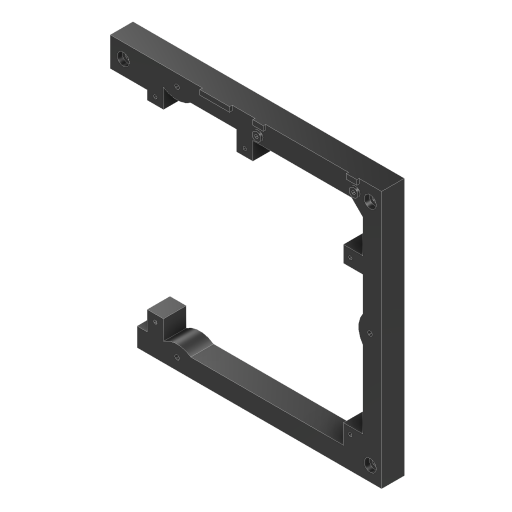
# Autodesk Inventor part: display_cover_part1
Saved by Autodesk Inventor 2023 (Build 270158000, 158)
## iProperties
Created: 2024-12-04
Part Number: display_cover_part1
Material: Polyacetátová pryskyřice, černá
Document SubType Name: Modeling
Designer: Marek
Density: 1.425 g/cm^3
Appearance: Lesklá – černá
Author: Marek
## iProperties of the stored document display_cover_part1_3D tisk.ipt
Created: 2024-12-18
Part Number: display_cover_part1_3D tisk
Material: Všeobecné
Document SubType Name: Modeling
Designer: Marek
Density: 1 g/cm^3
Appearance: Výchozí
Author: Marek
Autodesk Inventor part; units mm, degrees
ref_plane "YZ Plane" through (0, 0, 0) normal (1, 0, 0) x (0, 1, 0)
ref_plane "XZ Plane" through (0, 0, 0) normal (0, 1, 0) x (-1, 0, 0)
ref_plane "XY Plane" through (0, 0, 0) normal (0, 0, 1) x (1, 0, 0)
sketch "Náčrt1" plane through (0, 0, 0) normal (0, 0, 1) x (1, 0, 0)
  line L0 (0, 110.95) -> (0, -110.95) projected
  line L1 (-116.9, 0) -> (116.9, 0) projected
  line L2 (-83.5, 79.25) -> (83.5, 79.25)
  line L3 (83.5, -79.25) -> (-67, -79.25)
  line L4 (-83.5, 61.25) -> (-83.5, 79.25)
  line L5 (-65.5, 67.75) -> (4.25, 67.75)
  line L6 (72, 67.75) -> (72, 66.75) construction
  line L7 (-65.5, 67.75) -> (-65.5, 61.25)
  line L8 (-65.5, 61.25) -> (-83.5, 61.25)
  line L9 (-67, -67.75) -> (-67, -79.25)
  line L10 (-60.75, 65) -> (69.25, 65) construction
  line L11 (69.25, 65) -> (69.25, -65) construction
  line L12 (69.25, -65) -> (-60.75, -65) construction
  line L13 (-60.75, -65) -> (-60.75, 65) construction
  line L14 (-65.5, 61.25) -> (-60.75, 61.25)
  line L15 (-60.75, 61.25) -> (-60.75, 55.75)
  line L16 (-60.75, 55.75) -> (-50.75, 55.75)
  line L17 (-50.75, 55.75) -> (-50.75, 67.75)
  line L18 (4.25, 65) -> (4.25, 39.25) construction
  line L19 (4.25, 39.25) -> (69.25, 39.25) construction
  line L20 (4.25, 67.75) -> (4.25, 55.75)
  line L21 (4.25, 55.75) -> (-5.75, 55.75)
  line L22 (-5.75, 55.75) -> (-5.75, 67.75)
  line L23 (-67, -67.75) -> (72, -67.75)
  line L24 (83.5, 79.25) -> (83.5, -79.25)
  line L25 (-60.75, -67.75) -> (-60.75, -55.75)
  line L26 (-60.75, -55.75) -> (-50.75, -55.75)
  line L27 (-50.75, -55.75) -> (-50.75, -67.75)
  line L28 (72, 39.25) -> (60, 39.25)
  line L29 (60, 39.25) -> (60, 29.25)
  line L30 (60, 29.25) -> (72, 29.25)
  line L31 (60, -67.75) -> (60, -55.75)
  line L32 (60, -55.75) -> (72, -55.75)
  line L33 (4.25, 66.75) -> (72, 66.75)
  line L34 (4.25, 67.75) -> (72, 67.75) construction
  line L35 (72, 66.75) -> (72, -67.75)
  arc A0 (72, 8.415) -> (72, -8.415) centre (83.5, 0) ccw
  arc A1 (-50.765, 67.75) -> (-33.935, 67.75) centre (-42.35, 79.25) ccw
  arc A2 (-33.935, -67.75) -> (-50.765, -67.75) centre (-42.35, -79.25) ccw
  point P0 (0, 0)
  point P1 (-50.75, -67.739)
  point P2 (-50.75, 67.739)
  dimension "d1" = 158.5
  dimension "d3" = 11.5
  dimension "d7" = 18
  dimension "d8" = 18
  dimension "d15" = 130
  dimension "d16" = 130
  dimension "d17" = 2.75
  dimension "d19" = 10
  dimension "d20" = 40
  dimension "d21" = 65
  dimension "d22" = 12
  dimension "d23" = 10
  dimension "d24" = 12
  dimension "d28" = 67.75
  dimension "d29" = 83.5
  dimension "d30" = 11.5
  dimension "d31" = 83.5
  dimension "d32" = 67
  dimension "d33" = 12
  dimension "d34" = 10
  dimension "d35" = 50.75
  dimension "d36" = 12
  dimension "d37" = 10
  dimension "d38" = 29.25
  dimension "d41" = 12
  dimension "d42" = 12
  dimension "d45" = 12.5
  dimension "d118" = 28.5
  dimension "d121" = 42.35
  dimension "d122" = 42.35
  constraints: 68 end point, 28 point on line, 22 perpendicular, 6 horizontal, 6 point on circle, 3 centre point, 3 parallel, 2 midpoint, 2 tangent, 2 vertical, 2 other
  measures "d1" distance of L2.end L3.start
  measures "d3" distance between parallel lines of L2 L5
  measures "d7" distance between parallel lines of L4 L7
  measures "d8" distance between parallel lines of L8 L2
  measures "d15" distance between parallel lines of L10 L12
  measures "d16" distance between parallel lines of L11 L13
  measures "d17" distance between parallel lines of L6 L11
  measures "d19" distance of L15.end L16.end
  measures "d20" distance between parallel lines of L2 L19
  measures "d21" distance between parallel lines of L11 L18
  measures "d22" distance of L5.end L20.end
  measures "d23" distance of L20.end L21.end
  measures "d24" distance between parallel lines of L5 L16
  measures "d28" distance between parallel lines of L1 L23
  measures "d29" distance between parallel lines of L24 L0
  measures "d30" distance between parallel lines of L24 L6
  measures "d31" distance between parallel lines of L0 L4
  measures "d32" distance between parallel lines of L0 L9
  measures "d33" distance of L25.start L25.end
  measures "d34" distance of L25.end L26.end
  measures "d35" distance between parallel lines of L0 L27
  measures "d36" distance of L28.start L28.end
  measures "d37" distance of L28.end L29.end
  measures "d38" distance between parallel lines of L30 L1
  measures "d41" distance of L31.end L32.end
  measures "d42" distance of L31.start L31.end
  measures "d45" distance between parallel lines of L2 L33
  measures "d118" diameter of A0
  measures "d121" distance from line of L0 A1.centre
  measures "d122" distance from line of L0 A2.centre
extrude "Vysunutí1" add sketch "Náčrt1" along normal blind 14 contours L2 L24 L1 L35 L33 L20 L5 L0 | L0 L5 L7 L8 L4 L2 | L5 L20 L21 L0 | L0 L21 L22 L5 | L24 L3 L0 L23 L35 L1 | A1 L17 L5 | L7 L5 A1 L17 L16 L15 L14 | L35 A0 L1 | L1 A0 L35 | L0 L3 L9 L23 | L17 A1 L5 | L23 L27 A2 | L31 L32 L35 L23 | L35 L30 L29 L28 | L23 A2 L27 | A2 L23 L25 L26 L27
chamfer "Zkosení1" distance 7 angle 45 1 edges at (72, 66.75, 7)
sketch "Náčrt2" plane through (0, 0, 14) normal (0, 0, 1) x (1, 0, 0)
  line L0 (-116.9, 0) -> (116.9, 0) projected
  line L1 (0, 110.95) -> (0, -110.95) projected
  line L2 (-5.75, 55.75) -> (4.25, 55.75) projected
  line L3 (4.25, 55.75) -> (4.25, 66.75) projected
  line L4 (4.25, 66.75) -> (65, 66.75) projected
  line L5 (72, 59.75) -> (65, 66.75) projected
  line L6 (72, 59.75) -> (72, 39.25) projected
  line L7 (72, -55.75) -> (60, -55.75) projected
  line L8 (60, -55.75) -> (60, -67.75) projected
  line L9 (60, -67.75) -> (-33.935, -67.75) projected
  line L10 (-50.75, -67.739) -> (-50.75, -55.75) projected
  line L11 (-50.75, -55.75) -> (-60.75, -55.75) projected
  line L12 (-60.75, -55.75) -> (-60.75, -67.75) projected
  line L13 (-60.75, -67.75) -> (-67, -67.75) projected
  line L14 (-67, -67.75) -> (-67, -79.25) projected
  line L15 (-67, -79.25) -> (83.5, -79.25) projected
  line L16 (83.5, -79.25) -> (83.5, 79.25) projected
  line L17 (83.5, 79.25) -> (-83.5, 79.25) projected
  line L18 (-83.5, 79.25) -> (-83.5, 61.25) projected
  line L19 (-83.5, 61.25) -> (-60.75, 61.25) projected
  line L20 (-60.75, 61.25) -> (-60.75, 55.75) projected
  line L21 (-60.75, 55.75) -> (-50.75, 55.75) projected
  line L22 (-50.75, 55.75) -> (-50.75, 67.739) projected
  line L23 (-33.935, 67.75) -> (-5.75, 67.75) projected
  line L24 (-5.75, 67.75) -> (-5.75, 55.75) projected
  circle A0 centre (7.8, 71.3) radius 2.75
  circle A1 centre (67.5, 71.3) radius 2.75
  line L25 (72, 39.25) -> (60, 39.25) projected
  line L26 (60, 39.25) -> (60, 29.25) projected
  line L27 (60, 29.25) -> (72, 29.25) projected
  line L28 (72, 29.25) -> (72, 8.415) projected
  arc A2 (72, 8.415) -> (72, -8.415) centre (83.5, 0) ccw projected
  line L29 (72, -8.415) -> (72, -55.75) projected
  arc A3 (-33.935, -67.75) -> (-50.75, -67.739) centre (-42.35, -79.25) ccw projected
  arc A4 (-50.75, 67.739) -> (-33.935, 67.75) centre (-42.35, 79.25) ccw projected
  point P0 (0, 0)
  dimension "d49" = 16
  dimension "d50" = 7.95
  dimension "d52" = 7.95
  dimension "d53" = 59.7
  dimension "d61" = 5.5
  dimension "d62" = 5.5
  constraints: 2 centre point, 2 coincident
  measures "d49" distance from line of L16 point (67.5, 71.3)
  measures "d50" distance from line of point (67.5, 71.3) L17
  measures "d52" distance from line of L17 point (7.8, 71.3)
  measures "d53" distance of point (67.5, 71.3) point (7.8, 71.3)
  measures "d61" diameter of A0
  measures "d62" diameter of A1
extrude "Vysunutí2" add sketch "Náčrt2" along normal blind 1.35 contours A0 | A1
sketch "Náčrt3" plane through (7.8, 71.3, 15.35) normal (0, 0, 1) x (1, 0, 0)
  circle A0 centre (0, 0) radius 2.75 projected
  circle A1 centre (59.7, 0) radius 2.75 projected
  circle A2 centre (59.7, 0) radius 2.75 projected
  point P0 (-7.8, -71.3)
  constraints: 2 coincident
hole "Díra2" at (7.8, 71.3, 15.35) at (67.5, 71.3, 15.35) direction (0, 0, -1) diameter 2.1 depth 9 tip angle 118
sketch "Náčrt4" plane through (0, 0, 14) normal (0, 0, 1) x (1, 0, 0)
  circle A0 centre (67.5, 71.3) radius 2.75 projected
  circle A1 centre (7.8, 71.3) radius 2.75 projected
  line L0 (-5.75, 55.75) -> (4.25, 55.75) projected
  line L1 (4.25, 55.75) -> (4.25, 66.75) projected
  line L2 (4.25, 66.75) -> (65, 66.75) projected
  line L3 (72, 59.75) -> (65, 66.75) projected
  line L4 (72, 59.75) -> (72, 39.25) projected
  line L5 (72, -55.75) -> (60, -55.75) projected
  line L6 (60, -55.75) -> (60, -67.75) projected
  line L7 (60, -67.75) -> (-33.935, -67.75) projected
  line L8 (-50.75, -67.739) -> (-50.75, -55.75) projected
  line L9 (-50.75, -55.75) -> (-60.75, -55.75) projected
  line L10 (-60.75, -55.75) -> (-60.75, -67.75) projected
  line L11 (-60.75, -67.75) -> (-67, -67.75) projected
  line L12 (-67, -67.75) -> (-67, -79.25) projected
  line L13 (-67, -79.25) -> (83.5, -79.25) projected
  line L14 (83.5, -79.25) -> (83.5, 79.25) projected
  line L15 (83.5, 79.25) -> (-83.5, 79.25) projected
  line L16 (-83.5, 79.25) -> (-83.5, 61.25) projected
  line L17 (-83.5, 61.25) -> (-60.75, 61.25) projected
  line L18 (-60.75, 61.25) -> (-60.75, 55.75) projected
  line L19 (-60.75, 55.75) -> (-50.75, 55.75) projected
  line L20 (-50.75, 55.75) -> (-50.75, 67.739) projected
  line L21 (-33.935, 67.75) -> (-5.75, 67.75) projected
  line L22 (-5.75, 67.75) -> (-5.75, 55.75) projected
  line L23 (-116.9, 0) -> (116.9, 0) projected
  line L24 (0, 110.95) -> (0, -110.95) projected
  circle A2 centre (-75.5, 70.25) radius 3.75
  circle A3 centre (76.5, 70.25) radius 3.75
  circle A4 centre (76.5, -70.25) radius 3.75
  line L25 (72, 39.25) -> (60, 39.25) projected
  line L26 (60, 39.25) -> (60, 29.25) projected
  line L27 (60, 29.25) -> (72, 29.25) projected
  line L28 (72, 29.25) -> (72, 8.415) projected
  arc A5 (72, 8.415) -> (72, -8.415) centre (83.5, 0) ccw projected
  line L29 (72, -8.415) -> (72, -55.75) projected
  arc A6 (-33.935, -67.75) -> (-50.75, -67.739) centre (-42.35, -79.25) ccw projected
  arc A7 (-50.75, 67.739) -> (-33.935, 67.75) centre (-42.35, 79.25) ccw projected
  point P0 (0, 0)
  dimension "d72" = 7.5
  dimension "d73" = 7.5
  dimension "d74" = 7.5
  dimension "d75" = 9
  dimension "d76" = 8
  dimension "d77" = 7
  dimension "d78" = 9
  dimension "d79" = 7
  dimension "d80" = 9
  constraints: 3 centre point
  measures "d72" diameter of A2
  measures "d73" diameter of A3
  measures "d74" diameter of A4
  measures "d75" distance from line of A2.centre L15
  measures "d76" distance from line of A2.centre L16
  measures "d77" distance from line of L14 A3.centre
  measures "d78" distance from line of L15 A3.centre
  measures "d79" distance from line of L14 A4.centre
  measures "d80" distance from line of L13 A4.centre
extrude "Vysunutí3" cut sketch "Náčrt4" against normal blind 3 contours A2 | A3 | A4
sketch "Náčrt5" plane through (-75.5, 70.25, 11) normal (0, 0, 1) x (1, 0, 0)
  circle A0 centre (0, 0) radius 3.75 projected
  circle A1 centre (152, 0) radius 3.75 projected
  circle A2 centre (152, -140.5) radius 3.75 projected
  circle A3 centre (0, 0) radius 3.75 projected
  circle A4 centre (152, 0) radius 3.75 projected
  circle A5 centre (152, -140.5) radius 3.75 projected
  point P0 (75.5, -70.25)
  constraints: 3 coincident
hole "Díra3" at (-75.5, 70.25, 11) at (76.5, 70.25, 11) at (76.5, -70.25, 11) direction (0, 0, -1) diameter 3.7 end through all
sketch "Náčrt6" plane through (0, 0, 0) normal (0, 0, -1) x (-1, 0, 0)
  circle A0 centre (-76.5, 70.25) radius 1.85 projected
  circle A1 centre (75.5, 70.25) radius 1.85 projected
  circle A2 centre (-76.5, -70.25) radius 1.85 projected
  line L0 (5.75, 55.75) -> (-4.25, 55.75) projected
  line L1 (5.75, 67.75) -> (5.75, 55.75) projected
  line L2 (33.935, 67.75) -> (5.75, 67.75) projected
  line L3 (50.75, 55.75) -> (50.75, 67.739) projected
  line L4 (60.75, 55.75) -> (50.75, 55.75) projected
  line L5 (60.75, 61.25) -> (60.75, 55.75) projected
  line L6 (83.5, 61.25) -> (60.75, 61.25) projected
  line L7 (83.5, 79.25) -> (83.5, 61.25) projected
  line L8 (-83.5, 79.25) -> (83.5, 79.25) projected
  line L9 (-83.5, -79.25) -> (-83.5, 79.25) projected
  line L10 (67, -79.25) -> (-83.5, -79.25) projected
  line L11 (67, -67.75) -> (67, -79.25) projected
  line L12 (60.75, -67.75) -> (67, -67.75) projected
  line L13 (60.75, -55.75) -> (60.75, -67.75) projected
  line L14 (50.75, -55.75) -> (60.75, -55.75) projected
  line L15 (50.75, -67.739) -> (50.75, -55.75) projected
  line L16 (-60, -67.75) -> (33.935, -67.75) projected
  line L17 (-60, -55.75) -> (-60, -67.75) projected
  line L18 (-72, -55.75) -> (-60, -55.75) projected
  line L19 (-72, -8.415) -> (-72, -55.75) projected
  line L20 (-60, 29.25) -> (-72, 29.25) projected
  line L21 (-60, 39.25) -> (-60, 29.25) projected
  line L22 (-72, 39.25) -> (-60, 39.25) projected
  line L23 (-72, 59.75) -> (-72, 39.25) projected
  line L24 (-65, 66.75) -> (-72, 59.75) projected
  line L25 (-4.25, 66.75) -> (-65, 66.75) projected
  line L26 (-4.25, 55.75) -> (-4.25, 66.75) projected
  line L27 (-116.9, 0) -> (116.9, 0) projected
  line L28 (0, -110.95) -> (0, 110.95) projected
  arc A3 (-72, -8.415) -> (-72, 8.415) centre (-83.5, 0) ccw projected
  line L29 (-72, 29.25) -> (-72, 8.415) projected
  arc A4 (33.935, 67.75) -> (50.75, 67.739) centre (42.35, 79.25) ccw projected
  arc A5 (50.75, -67.739) -> (33.935, -67.75) centre (42.35, -79.25) ccw projected
  point P0 (0, 0)
  point P1 (-34.5, -72.45)
  dimension "d90" = 49
  dimension "d91" = 6.8
  measures "d90" distance from line of point (-34.5, -72.45) L9
  measures "d91" distance from line of L10 point (-34.5, -72.45)
hole "Díra4" at (34.5, -72.45, 0) direction (0, 0, 1) diameter 5 depth 4.3
sketch "Náčrt7" plane through (0, 0, 14) normal (0, 0, 1) x (1, 0, 0)
  circle A0 centre (76.5, -70.25) radius 3.75 projected
  circle A1 centre (76.5, 70.25) radius 3.75 projected
  circle A2 centre (-75.5, 70.25) radius 3.75 projected
  circle A3 centre (67.5, 71.3) radius 2.75 projected
  circle A4 centre (7.8, 71.3) radius 2.75 projected
  line L0 (-5.75, 55.75) -> (4.25, 55.75) projected
  line L1 (4.25, 55.75) -> (4.25, 66.75) projected
  line L2 (4.25, 66.75) -> (65, 66.75) projected
  line L3 (72, 59.75) -> (65, 66.75) projected
  line L4 (72, 59.75) -> (72, 39.25) projected
  line L5 (72, 39.25) -> (60, 39.25) projected
  line L6 (60, 39.25) -> (60, 29.25) projected
  line L7 (60, 29.25) -> (72, 29.25) projected
  line L8 (72, 29.25) -> (72, 8.415) projected
  line L9 (72, -55.75) -> (60, -55.75) projected
  line L10 (60, -55.75) -> (60, -67.75) projected
  line L11 (60, -67.75) -> (-33.935, -67.75) projected
  line L12 (-50.75, -67.739) -> (-50.75, -55.75) projected
  line L13 (-50.75, -55.75) -> (-60.75, -55.75) projected
  line L14 (-60.75, -55.75) -> (-60.75, -67.75) projected
  line L15 (-60.75, -67.75) -> (-67, -67.75) projected
  line L16 (-67, -67.75) -> (-67, -79.25) projected
  line L17 (-67, -79.25) -> (83.5, -79.25) projected
  line L18 (83.5, -79.25) -> (83.5, 79.25) projected
  line L19 (83.5, 79.25) -> (-83.5, 79.25) projected
  line L20 (-83.5, 79.25) -> (-83.5, 61.25) projected
  line L21 (-83.5, 61.25) -> (-60.75, 61.25) projected
  line L22 (-60.75, 61.25) -> (-60.75, 55.75) projected
  line L23 (-60.75, 55.75) -> (-50.75, 55.75) projected
  line L24 (-50.75, 55.75) -> (-50.75, 67.739) projected
  line L25 (-33.935, 67.75) -> (-5.75, 67.75) projected
  line L26 (-5.75, 67.75) -> (-5.75, 55.75) projected
  line L27 (-116.9, 0) -> (116.9, 0) projected
  line L28 (0, 110.95) -> (0, -110.95) projected
  arc A5 (72, 8.415) -> (72, -8.415) centre (83.5, 0) ccw projected
  line L29 (72, -8.415) -> (72, -55.75) projected
  arc A6 (-33.935, -67.75) -> (-50.75, -67.739) centre (-42.35, -79.25) ccw projected
  arc A7 (-50.75, 67.739) -> (-33.935, 67.75) centre (-42.35, 79.25) ccw projected
  point P0 (0, 0)
  point P1 (-55.75, 60)
  point P2 (-0.75, 60)
  point P3 (64.25, 34.25)
  point P4 (64.25, -60)
  point P5 (-55.75, -60)
  dimension "d99" = 5
  dimension "d100" = 7.75
  dimension "d101" = 7.75
  dimension "d102" = 5
  dimension "d103" = 7.75
  dimension "d104" = 5
  dimension "d106" = 7.75
  dimension "d107" = 7.75
  dimension "d108" = 7.75
  dimension "d110" = 5
  measures "d99" distance from line of point (-55.75, 60) L22
  measures "d100" distance from line of point (-55.75, 60) L25
  measures "d101" distance from line of point (-0.75, 60) L25
  measures "d102" distance from line of point (-0.75, 60) L26
  measures "d103" distance from line of L4 point (64.25, 34.25)
  measures "d104" distance from line of point (64.25, 34.25) L5
  measures "d106" distance from line of point (64.25, -60) L8
  measures "d107" distance from line of point (64.25, -60) L11
  measures "d108" distance from line of L11 point (-55.75, -60)
  measures "d110" distance from line of L14 point (-55.75, -60)
hole "Díra5" at (-55.75, 60, 14) at (-0.75, 60, 14) at (64.25, 34.25, 14) at (64.25, -60, 14) at (-55.75, -60, 14) direction (0, 0, -1) diameter 2.1 depth 16 tip angle 118
sketch "Náčrt8" plane through (0, 0, 14) normal (0, 0, 1) x (1, 0, 0)
  circle A0 centre (64.25, -60) radius 1.05 projected
  circle A1 centre (-0.75, 60) radius 1.05 projected
  circle A2 centre (-55.75, 60) radius 1.05 projected
  circle A3 centre (64.25, 34.25) radius 1.05 projected
  circle A4 centre (-55.75, -60) radius 1.05 projected
  circle A5 centre (76.5, -70.25) radius 3.75 projected
  circle A6 centre (76.5, 70.25) radius 3.75 projected
  circle A7 centre (-75.5, 70.25) radius 3.75 projected
  circle A8 centre (67.5, 71.3) radius 2.75 projected
  circle A9 centre (7.8, 71.3) radius 2.75 projected
  line L0 (-5.75, 55.75) -> (4.25, 55.75) projected
  line L1 (4.25, 55.75) -> (4.25, 66.75) projected
  line L2 (4.25, 66.75) -> (65, 66.75) projected
  line L3 (72, 59.75) -> (65, 66.75) projected
  line L4 (72, 59.75) -> (72, 39.25) projected
  line L5 (72, 39.25) -> (60, 39.25) projected
  line L6 (60, 39.25) -> (60, 29.25) projected
  line L7 (60, 29.25) -> (72, 29.25) projected
  line L8 (72, 29.25) -> (72, 8.415) projected
  arc A10 (72, 8.415) -> (72, -8.415) centre (83.5, 0) ccw projected
  line L9 (72, -8.415) -> (72, -55.75) projected
  line L10 (72, -55.75) -> (60, -55.75) projected
  line L11 (60, -55.75) -> (60, -67.75) projected
  line L12 (60, -67.75) -> (-33.935, -67.75) projected
  arc A11 (-33.935, -67.75) -> (-50.75, -67.739) centre (-42.35, -79.25) ccw projected
  line L13 (-50.75, -67.739) -> (-50.75, -55.75) projected
  line L14 (-50.75, -55.75) -> (-60.75, -55.75) projected
  line L15 (-60.75, -55.75) -> (-60.75, -67.75) projected
  line L16 (-60.75, -67.75) -> (-67, -67.75) projected
  line L17 (-67, -67.75) -> (-67, -79.25) projected
  line L18 (-67, -79.25) -> (83.5, -79.25) projected
  line L19 (83.5, -79.25) -> (83.5, 79.25) projected
  line L20 (83.5, 79.25) -> (-83.5, 79.25) projected
  line L21 (-83.5, 79.25) -> (-83.5, 61.25) projected
  line L22 (-83.5, 61.25) -> (-60.75, 61.25) projected
  line L23 (-60.75, 61.25) -> (-60.75, 55.75) projected
  line L24 (-60.75, 55.75) -> (-50.75, 55.75) projected
  line L25 (-50.75, 55.75) -> (-50.75, 67.739) projected
  arc A12 (-50.75, 67.739) -> (-33.935, 67.75) centre (-42.35, 79.25) ccw projected
  line L26 (-33.935, 67.75) -> (-5.75, 67.75) projected
  line L27 (-5.75, 67.75) -> (-5.75, 55.75) projected
  line L28 (0, 110.95) -> (0, -110.95) projected
  line L29 (-116.9, 0) -> (116.9, 0) projected
  line L30 (83.5, 79.25) -> (-83.5, 79.25) projected
  line L31 (5.6, 79.25) -> (69.6, 79.25)
  line L32 (69.6, 79.25) -> (69.6, 76.25)
  line L33 (69.6, 76.25) -> (5.6, 76.25)
  line L34 (5.6, 76.25) -> (5.6, 79.25)
  line L35 (12.1, 76.25) -> (5.6, 76.25)
  line L36 (5.6, 76.25) -> (5.6, 79.25)
  line L37 (5.6, 79.25) -> (12.1, 79.25)
  line L38 (12.1, 79.25) -> (12.1, 76.25)
  line L39 (69.6, 76.25) -> (63.1, 76.25)
  line L40 (63.1, 76.25) -> (63.1, 79.25)
  line L41 (63.1, 79.25) -> (69.6, 79.25)
  line L42 (69.6, 79.25) -> (69.6, 76.25)
  point P0 (0, 0)
  point P1 (63.1, 76.25)
  dimension "d123" = 64
  dimension "d124" = 3
  dimension "d125" = 13.9
  dimension "d126" = 6.5
  dimension "d127" = 6.5
  constraints: 24 end point, 6 parallel, 3 horizontal, 3 perpendicular, 3 point on line
  measures "d123" distance of L32.end L33.end
  measures "d124" distance of L31.end L32.end
  measures "d125" distance between parallel lines of L19 L32
  measures "d126" distance between parallel lines of L42 L40
  measures "d127" distance between parallel lines of L34 L38
extrude "Vysunutí4" add sketch "Náčrt8" along normal blind 1.35 contours L20 L38 L33 L34 | L20 L32 L33 L40
sketch "Náčrt9" plane through (0, 0, 14) normal (0, 0, 1) x (1, 0, 0)
  circle A0 centre (7.8, 71.3) radius 2.75 projected
  circle A1 centre (67.5, 71.3) radius 2.75 projected
  circle A2 centre (-75.5, 70.25) radius 3.75 projected
  circle A3 centre (76.5, 70.25) radius 3.75 projected
  circle A4 centre (76.5, -70.25) radius 3.75 projected
  circle A5 centre (-55.75, -60) radius 1.05 projected
  circle A6 centre (64.25, 34.25) radius 1.05 projected
  circle A7 centre (-55.75, 60) radius 1.05 projected
  circle A8 centre (-0.75, 60) radius 1.05 projected
  circle A9 centre (64.25, -60) radius 1.05 projected
  line L0 (69.6, 79.25) -> (69.6, 76.25) projected
  line L1 (69.6, 76.25) -> (63.1, 76.25) projected
  line L2 (63.1, 76.25) -> (63.1, 79.25) projected
  line L3 (63.1, 79.25) -> (12.1, 79.25) projected
  line L4 (12.1, 79.25) -> (12.1, 76.25) projected
  line L5 (12.1, 76.25) -> (5.6, 76.25) projected
  line L6 (5.6, 76.25) -> (5.6, 79.25) projected
  line L7 (5.6, 79.25) -> (-83.5, 79.25) projected
  line L8 (-83.5, 79.25) -> (-83.5, 61.25) projected
  line L9 (-83.5, 61.25) -> (-60.75, 61.25) projected
  line L10 (-60.75, 61.25) -> (-60.75, 55.75) projected
  line L11 (-60.75, 55.75) -> (-50.75, 55.75) projected
  line L12 (-50.75, 55.75) -> (-50.75, 67.739) projected
  arc A10 (-50.75, 67.739) -> (-33.935, 67.75) centre (-42.35, 79.25) ccw projected
  line L13 (-33.935, 67.75) -> (-5.75, 67.75) projected
  line L14 (-5.75, 67.75) -> (-5.75, 55.75) projected
  line L15 (-5.75, 55.75) -> (4.25, 55.75) projected
  line L16 (4.25, 55.75) -> (4.25, 66.75) projected
  line L17 (4.25, 66.75) -> (65, 66.75) projected
  line L18 (72, 59.75) -> (65, 66.75) projected
  line L19 (72, 59.75) -> (72, 39.25) projected
  line L20 (72, 39.25) -> (60, 39.25) projected
  line L21 (60, 39.25) -> (60, 29.25) projected
  line L22 (60, 29.25) -> (72, 29.25) projected
  line L23 (72, 29.25) -> (72, 8.415) projected
  arc A11 (72, 8.415) -> (72, -8.415) centre (83.5, 0) ccw projected
  line L24 (72, -8.415) -> (72, -55.75) projected
  line L25 (72, -55.75) -> (60, -55.75) projected
  line L26 (60, -55.75) -> (60, -67.75) projected
  line L27 (60, -67.75) -> (-33.935, -67.75) projected
  arc A12 (-33.935, -67.75) -> (-50.75, -67.739) centre (-42.35, -79.25) ccw projected
  line L28 (-50.75, -67.739) -> (-50.75, -55.75) projected
  line L29 (-50.75, -55.75) -> (-60.75, -55.75) projected
  line L30 (-60.75, -55.75) -> (-60.75, -67.75) projected
  line L31 (-60.75, -67.75) -> (-67, -67.75) projected
  line L32 (-67, -67.75) -> (-67, -79.25) projected
  line L33 (-67, -79.25) -> (83.5, -79.25) projected
  line L34 (83.5, -79.25) -> (83.5, 79.25) projected
  line L35 (83.5, 79.25) -> (69.6, 79.25) projected
  line L36 (83.5, 79.25) -> (-83.5, 79.25) projected
  line L37 (-26.8, 79.25) -> (-8.5, 79.25)
  line L38 (-8.5, 79.25) -> (-8.5, 76.25)
  line L39 (-8.5, 76.25) -> (-26.8, 76.25)
  line L40 (-26.8, 76.25) -> (-26.8, 79.25)
  point P0 (0, 0)
  dimension "d130" = 92
  dimension "d131" = 110.3
  dimension "d132" = 3
  constraints: 8 end point, 2 parallel, 1 horizontal, 1 perpendicular, 1 point on line
  measures "d130" distance between parallel lines of L34 L38
  measures "d131" distance between parallel lines of L34 L40
  measures "d132" distance between parallel lines of L36 L39
extrude "Vysunutí5" add sketch "Náčrt9" along normal blind 1.6 contours L38 L39 L40 L7
sketch "Náčrt10" plane through (0, 0, 14) normal (0, 0, 1) x (1, 0, 0)
  line L0 (-26.8, 76.25) -> (-8.5, 76.25) projected
  line L1 (-26.8, 76.25) -> (-26.8, 79.25) projected
  line L2 (-26.8, 79.25) -> (-83.5, 79.25) projected
  line L3 (-83.5, 79.25) -> (-83.5, 61.25) projected
  line L4 (-83.5, 61.25) -> (-60.75, 61.25) projected
  line L5 (-60.75, 61.25) -> (-60.75, 55.75) projected
  line L6 (-60.75, 55.75) -> (-50.75, 55.75) projected
  line L7 (-50.75, 55.75) -> (-50.75, 67.739) projected
  arc A0 (-50.75, 67.739) -> (-33.935, 67.75) centre (-42.35, 79.25) ccw projected
  line L8 (-33.935, 67.75) -> (-5.75, 67.75) projected
  line L9 (-5.75, 67.75) -> (-5.75, 55.75) projected
  line L10 (-5.75, 55.75) -> (4.25, 55.75) projected
  line L11 (4.25, 55.75) -> (4.25, 66.75) projected
  line L12 (4.25, 66.75) -> (65, 66.75) projected
  line L13 (72, 59.75) -> (65, 66.75) projected
  line L14 (72, 59.75) -> (72, 39.25) projected
  line L15 (72, 39.25) -> (60, 39.25) projected
  line L16 (60, 39.25) -> (60, 29.25) projected
  line L17 (60, 29.25) -> (72, 29.25) projected
  line L18 (72, 29.25) -> (72, 8.415) projected
  arc A1 (72, 8.415) -> (72, -8.415) centre (83.5, 0) ccw projected
  line L19 (72, -8.415) -> (72, -55.75) projected
  line L20 (72, -55.75) -> (60, -55.75) projected
  line L21 (60, -55.75) -> (60, -67.75) projected
  line L22 (60, -67.75) -> (-33.935, -67.75) projected
  arc A2 (-33.935, -67.75) -> (-50.75, -67.739) centre (-42.35, -79.25) ccw projected
  line L23 (-50.75, -67.739) -> (-50.75, -55.75) projected
  line L24 (-50.75, -55.75) -> (-60.75, -55.75) projected
  line L25 (-60.75, -55.75) -> (-60.75, -67.75) projected
  line L26 (-60.75, -67.75) -> (-67, -67.75) projected
  line L27 (-67, -67.75) -> (-67, -79.25) projected
  line L28 (-67, -79.25) -> (83.5, -79.25) projected
  line L29 (83.5, -79.25) -> (83.5, 79.25) projected
  line L30 (83.5, 79.25) -> (69.6, 79.25) projected
  line L31 (69.6, 79.25) -> (69.6, 76.25) projected
  line L32 (69.6, 76.25) -> (63.1, 76.25) projected
  line L33 (63.1, 76.25) -> (63.1, 79.25) projected
  line L34 (63.1, 79.25) -> (12.1, 79.25) projected
  line L35 (12.1, 79.25) -> (12.1, 76.25) projected
  line L36 (12.1, 76.25) -> (5.6, 76.25) projected
  line L37 (5.6, 76.25) -> (5.6, 79.25) projected
  line L38 (5.6, 79.25) -> (-8.5, 79.25) projected
  line L39 (-8.5, 79.25) -> (-8.5, 76.25) projected
  line L40 (-8.5, 76.25) -> (-26.8, 76.25) projected
  circle A3 centre (7.8, 71.3) radius 2.75 projected
  circle A4 centre (67.5, 71.3) radius 2.75 projected
  circle A5 centre (-75.5, 70.25) radius 3.75 projected
  circle A6 centre (76.5, 70.25) radius 3.75 projected
  circle A7 centre (76.5, -70.25) radius 3.75 projected
  circle A8 centre (-55.75, -60) radius 1.05 projected
  circle A9 centre (64.25, 34.25) radius 1.05 projected
  circle A10 centre (-55.75, 60) radius 1.05 projected
  circle A11 centre (-0.75, 60) radius 1.05 projected
  circle A12 centre (64.25, -60) radius 1.05 projected
  line L41 (0, 110.95) -> (0, -110.95) projected
  line L42 (-116.9, 0) -> (116.9, 0) projected
  point P0 (0, 0)
  point P1 (-42.3407, 72.125)
  point P2 (76.375, 0)
  point P3 (-42.3407, -72.125)
  dimension "d135" = 7.125
  dimension "d136" = 42.3407
  dimension "d137" = 7.125
  dimension "d138" = 42.3407
  dimension "d139" = 7.125
  constraints: 1 point on line
  measures "d135" distance from line of L28 point (-42.341, -72.125)
  measures "d136" distance from line of L41 point (-42.341, -72.125)
  measures "d137" distance from line of L2 point (-42.341, 72.125)
  measures "d138" distance from line of L41 point (-42.341, 72.125)
  measures "d139" distance from line of L29 point (76.375, 0)
hole "Díra6" at (-42.3407, 72.125, 14) at (76.375, 0, 14) at (-42.3407, -72.125, 14) direction (0, 0, -1) diameter 2.8 depth 14
